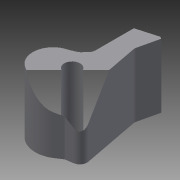
# Autodesk Inventor part: ExtruderSatoerCam
Saved by Autodesk Inventor 2015 SP1 (Build 190203100, 203)
## iProperties
Created: 2015-05-03
Part Number: ExtruderSatoerCam
Material: Generic
Document SubType Name: Modeling
Designer: Jack
Density: 1 g/cm^3
Appearance: Default
Author: Jack
Autodesk Inventor part; units mm, degrees
ref_plane "YZ Plane" through (0, 0, 0) normal (1, 0, 0) x (0, 1, 0)
ref_plane "XZ Plane" through (0, 0, 0) normal (0, 1, 0) x (-1, 0, 0)
ref_plane "XY Plane" through (0, 0, 0) normal (0, 0, 1) x (1, 0, 0)
sketch "Sketch1" plane through (0, 0, 0) normal (0, 0, 1) x (1, 0, 0)
  line L0 (0, 0) -> (89.1946, 0) construction
  line L1 (89.1946, 0) -> (89.1946, -45.0628) construction
  line L2 (89.1946, -45.0628) -> (0, -45.0628) construction
  line L3 (0, -45.0628) -> (0, 0) construction
  line L4 (45.8, -14.477) -> (45.8, -2.9)
  line L5 (45.8, -2.9) -> (51.6, -1.25)
  line L6 (51.6, -1.25) -> (52.2, -1.62)
  line L7 (52.2, -1.62) -> (50.8, -7.72)
  line L8 (50.8, -7.72) -> (54.3, -25.9)
  line L9 (48, -27.85) -> (50, -26.55)
  line L10 (50, -26.55) -> (54.3, -25.9)
  arc A0 (38.5438, -26.3298) -> (48, -27.85) centre (44.1464, -21.65) ccw
  arc A1 (41.9, -17.327) -> (38.5438, -26.3298) centre (43.0964, -22.9) ccw
  line L11 (43.9, -16.477) -> (45.8, -14.477)
  line L12 (41.9, -17.327) -> (43.9, -16.477)
  dimension "d26" = 45.8
  dimension "d27" = 2.9
  dimension "d29" = 5.8
  dimension "d30" = 1.65
  dimension "d31" = 0.6
  dimension "d32" = 0.37
  dimension "d33" = 6.1
  dimension "d34" = 1.4
  dimension "d36" = 3.5
  dimension "d37" = 0.65
  dimension "d38" = 4.3
  dimension "d39" = 1.3
  dimension "d40" = 2
  dimension "d41" = 7.3
  dimension "d42" = 5.7
  dimension "d44" = 1.05
  dimension "d45" = 1.25
  dimension "d46" = 20
  dimension "d47" = 0.85
  dimension "d48" = 2
  dimension "d49" = 2
  dimension "d50" = 1.9
  dimension "d65" = 23
  constraints: 20 end point, 4 point on circle, 2 centre point, 2 horizontal, 1 vertical, 4 other
  measures "d26" horizontal distance of point (0, 0) L4.end
  measures "d27" vertical distance of L4.end L0.start
  measures "d29" horizontal distance of L5.end L4.end
  measures "d30" vertical distance of L5.end L4.end
  measures "d31" horizontal distance of L6.end L5.end
  measures "d32" vertical distance of L5.end L6.end
  measures "d33" vertical distance of L7.end L6.end
  measures "d34" horizontal distance of L7.end L6.end
  measures "d36" horizontal distance of L8.end L7.end
  measures "d37" vertical distance of L8.end L9.end
  measures "d38" horizontal distance of L8.end L9.end
  measures "d39" vertical distance of L9.start L9.end
  measures "d40" horizontal distance of L9.start L9.end
  measures "d41" radius of A0
  measures "d42" radius of A1
  measures "d44" horizontal distance of A0.centre A1.centre
  measures "d45" vertical distance of A0.centre A1.centre
  measures "d46" vertical distance of L4.end A1.centre
  measures "d47" vertical distance of L11.start L12.start
  measures "d48" horizontal distance of L12.start L11.start
  measures "d49" vertical distance of L4.start L11.start
  measures "d50" horizontal distance of L4.start L11.start
  measures "d65" vertical distance of L8.end L4.end
extrude "Extrusion2" add sketch "Sketch1" along normal blind 18
fillet "Fillet1" radius 2 4 edges at (54.3, -25.9, 9) (45.8, -14.477, 9) (43.9, -16.477, 9) (50.8, -7.72, 9)
sketch "Sketch3" plane through (0, 0, 18) normal (0, 0, 1) x (1, 0, 0)
  line L0 (45.8, -2.9) -> (45.8, -13.6784) projected
  point P0 (51.6, -1.25)
  point P1 (0, 0)
  point P2 (46.8, -22.25)
  dimension "d54" = 1
  dimension "d55" = 21
  measures "d54" distance from line of L0 point (46.8, -22.25)
  measures "d55" vertical distance of point (46.8, -22.25) point (51.6, -1.25)
hole "Hole1" at (46.8, -22.25, 18) direction (0, 0, -1) diameter 4.5 end through all
body "Solid2"
